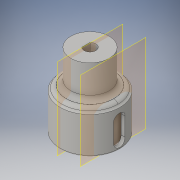
# Autodesk Inventor part: Autofeeder part 1
Saved by Autodesk Inventor 2016 (Build 200138000, 138)
## iProperties
Created: 2016-12-02
Part Number: Autofeeder part 1
Material: Generic
Document SubType Name: Modeling
Designer: Student
Density: 1 g/cm^3
Appearance: Default
Author: Student
Autodesk Inventor part; units mm, degrees
ref_plane "XZ Plane" through (0, 0, 0) normal (0, 1, 0) x (-1, 0, 0)
ref_plane "XY Plane" through (0, 0, 0) normal (0, 0, 1) x (1, 0, 0)
sketch "Sketch1" plane through (0, 0, 0) normal (0, 1, 0) x (-1, 0, 0)
  circle A0 centre (0, 0) radius 3.2318
  line L0 (2.28, 2.2905) -> (2.28, -2.2905)
  circle A1 centre (0, 0) radius 10.5918
  dimension "d2" = 5.5118
  dimension "d3" = 21.1836
  constraints: 2 centre point, 2 coincident, 2 end point, 2 point on circle, 1 vertical
  measures "d3" diameter of A1
extrude "Extrusion1" add sketch "Sketch1" along normal blind 18.034 contours A0 L0 | A1 picked at (2.4147, -0.6)
sketch "Sketch2" plane through (0, 0, 0) normal (0, -1, 0) x (1, 0, 0)
  circle A0 centre (0, 0) radius 15.24
  dimension "d6" = 30.48
  constraints: 1 centre point, 1 coincident
  measures "d6" diameter of A0
extrude "Extrusion2" add sketch "Sketch2" along normal blind 2.54
sketch "Sketch3" plane through (0, -2.54, 0) normal (0, -1, 0) x (1, 0, 0)
  circle A0 centre (0, 0) radius 14.351
  circle A1 centre (0, 0) radius 16.4291
  dimension "d9" = 28.702
  constraints: 2 centre point, 2 coincident
  measures "d9" diameter of A0
extrude "Extrusion3" add sketch "Sketch3" along normal blind 20.32
fillet "Fillet3" radius 2.54 1 edges at (10.5918, 0, 0)
fillet "Fillet4" radius 2.54 1 edges at (-15.24, -2.54, 0)
fillet "Fillet5" radius 2.54 1 edges at (-15.24, 0, 0)
ref_plane "Work Plane1" through (12.7, 0, 0) normal (1, 0, 0) x (0, 1, 0)
sketch "Sketch6" plane through (12.7, 0, 0) normal (1, 0, 0) x (0, 1, 0)
  arc A0 (-8.3185, -1.27) -> (-8.3185, 1.27) centre (-8.3185, 0) ccw construction
  arc A1 (-18.4785, 1.27) -> (-18.4785, -1.27) centre (-18.4785, 0) ccw construction
  line L0 (-18.4785, 1.27) -> (-8.3185, 1.27) construction
  line L1 (-8.3185, -1.27) -> (-18.4785, -1.27) construction
  arc A2 (-8.3185, -3.175) -> (-8.3185, 3.175) centre (-8.3185, 0) ccw
  line L2 (-8.3185, -3.175) -> (-18.4785, -3.175)
  arc A3 (-18.4785, 3.175) -> (-18.4785, -3.175) centre (-18.4785, 0) ccw
  line L3 (-18.4785, 3.175) -> (-8.3185, 3.175)
  point P0 (0, 0)
  dimension "d34" = 3.175
  constraints: 8 end point, 8 point on circle, 4 centre point, 3 other
  measures "d34" distance from line of A1.centre L3
extrude "Extrusion6" cut sketch "Sketch6" along normal blind 25.4
mirror "Mirror1" about plane through (0, 0, 0) normal (1, 0, 0) of "Extrusion6"
fillet "Fillet10" radius 0.762 1 edges at (-16.4291, -22.86, 0)
sketch "Sketch7" plane through (0, -2.54, 0) normal (0, -1, 0) x (1, 0, 0)
  circle A0 centre (0, 0) radius 12.7
  dimension "d40" = 25.4
  constraints: 1 centre point, 1 coincident
  measures "d40" diameter of A0
extrude "Extrusion7" add sketch "Sketch7" along normal blind 20.32
sketch "Sketch8" plane through (0, -22.86, 0) normal (0, -1, 0) x (1, 0, 0)
  line L0 (-0.4572, 8.89) -> (0.4572, 8.89)
  line L1 (0.4572, 8.89) -> (0.4572, -8.89)
  line L2 (0.4572, -8.89) -> (-0.4572, -8.89)
  line L3 (-0.4572, -8.89) -> (-0.4572, 8.89)
  line L4 (-0.4572, 8.89) -> (0.4572, -8.89) construction
  line L5 (0.4572, 8.89) -> (-0.4572, -8.89) construction
  point P0 (0, 0)
  dimension "d43" = 0.9144
  dimension "d44" = 17.78
  constraints: 12 end point, 2 midpoint, 2 parallel, 1 horizontal, 1 perpendicular
  measures "d43" distance of L1.end L2.end
  measures "d44" distance of L0.end L1.end
extrude "Extrusion8" cut sketch "Sketch8" against normal blind 20.32
body "Solid1"
